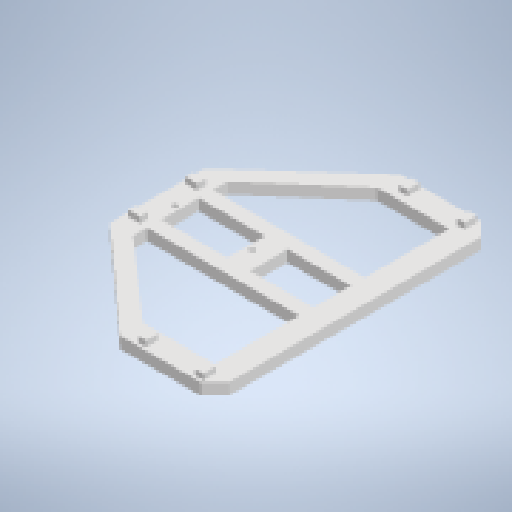
# Autodesk Inventor part: TopServoMount
Saved by Autodesk Inventor 2024.2 (Build 282272000, 272)
## iProperties
Created: 2024-04-02
Part Number: TopServoMount
Material: Generic
Document SubType Name: Modeling
Designer: ringl
Density: 1 g/cm^3
Appearance: Default
Author: ringl
Autodesk Inventor part; units mm, degrees
ref_plane "YZ Plane" through (0, 0, 0) normal (1, 0, 0) x (0, 1, 0)
ref_plane "XZ Plane" through (0, 0, 0) normal (0, 1, 0) x (-1, 0, 0)
ref_plane "XY Plane" through (0, 0, 0) normal (0, 0, 1) x (1, 0, 0)
sketch "Sketch1" plane through (0, 0, 0) normal (0, 1, 0) x (-1, 0, 0)
  line L0 (0, -59.5) -> (33, -59.5)
  line L1 (69, -27.15) -> (69, 5.85)
  line L2 (33, 38.2) -> (69, 5.85)
  line L3 (33, -59.5) -> (69, -27.15)
  line L4 (61, -27.15) -> (33, -51.5)
  line L5 (0, 38.2) -> (33, 38.2)
  line L6 (0, -59.5) -> (0, 38.2)
  line L7 (33, 30.2) -> (8, 30.2)
  line L8 (8, -51.5) -> (33, -51.5)
  line L9 (8, 30.2) -> (8, 0.85)
  line L10 (61, -17.15) -> (61, -4.15)
  line L11 (8, -4.15) -> (8, -17.15)
  line L12 (8, -22.15) -> (8, -51.5)
  line L13 (38, -17.15) -> (38, -4.15)
  line L14 (30, -4.15) -> (30, -17.15)
  line L15 (8, -17.15) -> (30, -17.15)
  line L16 (38, -17.15) -> (61, -17.15)
  line L17 (61, -4.15) -> (38, -4.15)
  line L18 (30, -4.15) -> (8, -4.15)
  line L19 (33, 30.2) -> (61, 5.85)
  line L20 (61, -27.15) -> (61, -22.15)
  line L21 (61, -22.15) -> (8, -22.15)
  line L22 (61, 5.85) -> (61, 0.85)
  line L23 (61, 0.85) -> (8, 0.85)
  point P0 (0, 0)
  point P1 (38, -10.65)
  dimension "d59" = 33
  dimension "d85" = 33
  dimension "d95" = 8
  dimension "d97" = 97.7
  dimension "d99" = 59.5
  dimension "d102" = 69
  dimension "d103" = 8
  dimension "d105" = 23
  dimension "d106" = 13
  dimension "d112" = 8
  dimension "d113" = 8
  dimension "d114" = 8
  dimension "d115" = 8
  dimension "d119" = 8
  dimension "d120" = 13
  dimension "d122" = 8
  dimension "d138" = 5
  dimension "d139" = 5
  dimension "d141" = 5
  dimension "d157" = 5
  dimension "d158" = 48.85
  constraints: 48 end point, 6 horizontal, 5 perpendicular, 4 vertical, 4 vertical alignment, 3 horizontal alignment, 1 midpoint, 1 parallel, 1 point on line
  measures "d59" distance of L0.start L0.end
  measures "d85" distance of L1.start L1.end
  measures "d95" distance of L0.end L4.end
  measures "d97" distance between parallel lines of L0 L5
  measures "d99" distance from line of point (0, 0) L0
  measures "d102" distance between parallel lines of L6 L1
  measures "d103" distance between parallel lines of L5 L7
  measures "d105" distance between parallel lines of L10 L13
  measures "d106" distance of L10.start L10.end
  measures "d112" distance of L1.start L4.start
  measures "d113" distance of L1.end L19.end
  measures "d114" distance from line of point (38, -10.65) L14
  measures "d115" distance between parallel lines of L6 L11
  measures "d119" distance between parallel lines of L1 L10
  measures "d120" distance of L14.start L14.end
  measures "d122" distance between parallel lines of L6 L9
  measures "d138" distance between parallel lines of L17 L23
  measures "d139" distance between parallel lines of L21 L15
  measures "d141" distance of L4.start L20.end
  measures "d157" distance between parallel lines of L23 L18
  measures "d158" distance from line of L5 point (38, -10.65)
extrude "Extrusion1" add sketch "Sketch1" along normal blind 4
sketch "Sketch4" plane through (0, 4, 0) normal (0, 1, 0) x (1, 0, 0)
  line L0 (-27.9, -37.1) -> (-25.1, -37.1)
  line L1 (-25.1, -37.1) -> (-25.1, -32.8)
  line L2 (-25.1, -32.8) -> (-27.9, -32.8)
  line L3 (-27.9, -32.8) -> (-27.9, -37.1)
  line L4 (-5.1, -32.8) -> (-7.9, -32.8)
  line L5 (-7.9, -32.8) -> (-7.9, -37.1)
  line L6 (-7.9, -37.1) -> (-5.1, -37.1)
  line L7 (-5.1, -37.1) -> (-5.1, -32.8)
  line L8 (-27.9, 54.1) -> (-25.1, 54.1)
  line L9 (-25.1, 54.1) -> (-25.1, 58.4)
  line L10 (-25.1, 58.4) -> (-27.9, 58.4)
  line L11 (-27.9, 58.4) -> (-27.9, 54.1)
  line L12 (-5.1, 54.1) -> (-7.9, 54.1)
  line L13 (-7.9, 54.1) -> (-7.9, 58.4)
  line L14 (-7.9, 58.4) -> (-5.1, 58.4)
  line L15 (-5.1, 58.4) -> (-5.1, 54.1)
  line L16 (0, 59.5) -> (-33, 59.5) projected
  line L17 (0, -38.2) -> (0, 59.5) projected
  line L18 (-33, -38.2) -> (0, -38.2) projected
  line L19 (-63.6, -0.75) -> (-67.9, -0.75)
  line L20 (-67.9, -0.75) -> (-67.9, 2.05)
  line L21 (-67.9, 2.05) -> (-63.6, 2.05)
  line L22 (-63.6, 2.05) -> (-63.6, -0.75)
  line L23 (-63.6, 19.25) -> (-67.9, 19.25)
  line L24 (-67.9, 19.25) -> (-67.9, 22.05)
  line L25 (-67.9, 22.05) -> (-63.6, 22.05)
  line L26 (-63.6, 22.05) -> (-63.6, 19.25)
  line L27 (-69, 27.15) -> (-69, -5.85) projected
  point P0 (0, 0)
  dimension "d60" = 4.3
  dimension "d63" = 2.8
  dimension "d64" = 2.8
  dimension "d66" = 17.2
  dimension "d67" = 4.3
  dimension "d68" = 1.1
  dimension "d133" = 5.1
  dimension "d134" = 1.1
  dimension "d150" = 4.3
  dimension "d151" = 2.8
  dimension "d152" = 4.3
  dimension "d153" = 2.8
  dimension "d154" = 17.2
  dimension "d155" = 1.1
  dimension "d156" = 5.1
  constraints: 48 end point, 12 parallel, 9 point on line, 6 horizontal, 6 perpendicular
  measures "d60" distance of L0.end L1.end
  measures "d63" distance of L5.end L6.end
  measures "d64" distance of L0.start L0.end
  measures "d66" distance between parallel lines of L1 L5
  measures "d67" distance of L14.end L12.start
  measures "d68" distance between parallel lines of L16 L14
  measures "d133" distance between parallel lines of L17 L7
  measures "d134" distance between parallel lines of L6 L18
  measures "d150" distance of L20.end L21.end
  measures "d151" distance of L19.end L20.end
  measures "d152" distance of L24.end L25.end
  measures "d153" distance of L23.end L24.end
  measures "d154" distance between parallel lines of L23 L21
  measures "d155" distance between parallel lines of L27 L20
  measures "d156" distance from line of L27.end L19
extrude "Extrusion5" add sketch "Sketch4" along normal blind 2
chamfer "Chamfer6" distance 5 angle 45 2 edges at (0, 2, -59.5) (0, 2, 38.2)
sketch "Sketch5" plane through (0, 0, 0) normal (0, -1, 0) x (1, 0, 0)
  circle A0 centre (-63, -10.65) radius 1
  circle A1 centre (-36, -10.65) radius 1
  line L0 (-38, -17.15) -> (-38, -4.15) projected
  line L1 (-61, -4.15) -> (-61, -17.15) projected
  line L2 (-38, -4.15) -> (-61, -4.15) projected
  line L3 (-61, -17.15) -> (-38, -17.15) projected
  point P0 (0, 0)
  dimension "d142" = 2
  dimension "d143" = 2
  dimension "d144" = 2
  dimension "d145" = 2
  dimension "d146" = 6.5
  dimension "d147" = 6.5
  constraints: 2 centre point
  measures "d142" diameter of A0
  measures "d143" diameter of A1
  measures "d144" distance from line of L0 A1.centre
  measures "d145" distance from line of A0.centre L1
  measures "d146" distance from line of L2 A0.centre
  measures "d147" distance from line of L3 A1.centre
extrude "Extrusion7" cut sketch "Sketch5" against normal blind 9 contours A0 | A1
body "Solid1"
